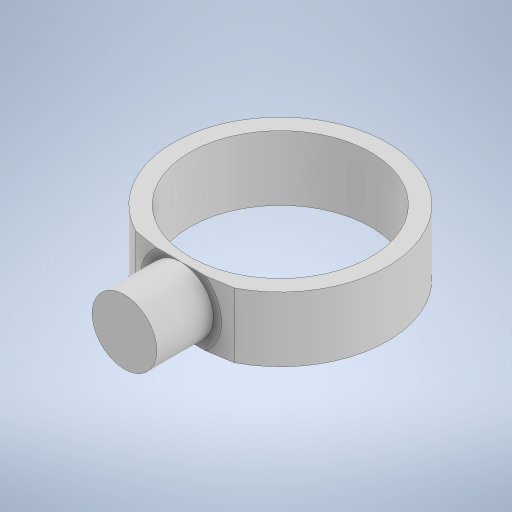
# Autodesk Inventor part: borde libre
Saved by Autodesk Inventor 2024 (Build 280153000, 153)
## iProperties
Created: 2024-04-03
Part Number: borde libre
Material: Generic
Document SubType Name: Modeling
Designer: compu
Density: 1 g/cm^3
Appearance: Default
Author: compu
Autodesk Inventor part; units mm, degrees
ref_plane "YZ Plane" through (0, 0, 0) normal (1, 0, 0) x (0, 1, 0)
ref_plane "XZ Plane" through (0, 0, 0) normal (0, 1, 0) x (-1, 0, 0)
ref_plane "XY Plane" through (0, 0, 0) normal (0, 0, 1) x (1, 0, 0)
sketch "Sketch1" plane through (0, 0, 0) normal (0, 1, 0) x (-1, 0, 0)
  line L0 (0, -18.55) -> (0, 18.55) projected
  line L1 (18.55, 0) -> (-18.55, 0) projected
  circle A0 centre (0, 0) radius 4
  circle A1 centre (0, 0) radius 11.2
  circle A2 centre (0, 0) radius 13.25
  line L2 (5, 12.2704) -> (-5, 12.2704)
  line L3 (6.0844, 11.7704) -> (-6.0844, 11.7704)
  dimension "d0" = 8
  dimension "d1" = 22.4
  dimension "d2" = 26.5
  dimension "d3" = 10
  dimension "d4" = 2.05
  dimension "d5" = 0.5
  constraints: 4 end point, 4 point on circle, 3 centre point, 3 coincident, 1 horizontal, 1 parallel
  measures "d0" diameter of A0
  measures "d1" diameter of A1
  measures "d2" diameter of A2
  measures "d3" distance of L2.start L2.end
  measures "d4" radial gap between concentric circles of A2 A1
  measures "d5" distance between parallel lines of L3 L2
extrude "Extrusion1" add sketch "Sketch1" along normal blind 8 contours A2 L1 A1 L0 | L0 A1 L1 A2 | A2 L3 L0 A1 L1 | L1 A1 L0 L3 A2
ref_plane "Work Plane1" through (6.0844, 0, 11.7704) normal (0, 0, 1) x (1, 0, 0)
sketch "Sketch2" plane through (6.0844, 0, 11.7704) normal (0, 0, 1) x (1, 0, 0)
  line L0 (-12.1689, 0) -> (0, 0) projected
  line L1 (0, 0) -> (0, 8) projected
  line L2 (-12.1689, 8) -> (0, 8) projected
  line L3 (-12.1689, 0) -> (-12.1689, 8) projected
  line L4 (-6.0844, -4.4) -> (-6.0844, 12.4) projected
  circle A0 centre (-6.0844, 4) radius 5
  point P0 (-6.0844, 0)
  point P1 (-9.0844, 8)
  point P2 (-9.0844, 0)
  point P3 (-3.0844, 0)
  point P4 (-3.0844, 8)
  dimension "d8" = 10
  dimension "d9" = 4
  constraints: 1 centre point, 1 midpoint
  measures "d8" diameter of A0
  measures "d9" distance from line of L0 A0.centre
extrude "Extrusion2" add sketch "Sketch2" along normal blind 0.5 contours A0 L2 L4 L0 | L4 L2 A0 L0
sketch "Sketch3" plane through (6.0844, 0, 12.2704) normal (0, 0, 1) x (1, 0, 0)
  line L0 (-9.0844, 0) -> (-3.0844, 0) projected
  arc A0 (-3.0844, 0) -> (-3.0844, 8) centre (-6.0844, 4) ccw projected
  line L1 (-3.0844, 8) -> (-9.0844, 8) projected
  arc A1 (-9.0844, 8) -> (-9.0844, 0) centre (-6.0844, 4) ccw projected
  circle A2 centre (-6.0844, 4) radius 4
  point P0 (-6.0844, 0)
  point P1 (-6.0844, 8)
  point P2 (-9.7017, 7)
  point P3 (-6.0844, 0)
  point P4 (-5.8287, 0)
  dimension "d12" = 8
  constraints: 1 centre point, 1 coincident
  measures "d12" diameter of A2
extrude "Extrusion3" add sketch "Sketch3" along normal blind 7 contours A2
loft "Loft1" add section 1 edges at (-4, 4, 12.2704) (-1.5, 8, 12.2704) (-5, 4, 12.2704) (-1.5, 0, 12.2704) section 2 edges at (-5, 4, 11.7704) (-4.5422, 8, 11.7704) (-6.0844, 4, 11.7704) (-4.5422, 0, 11.7704)
loft "Loft2" add section 1 edges at (2.8284, 6.8284, 12.2704) (2.8284, 1.1716, 12.2704) (1.5, 0, 12.2704) (5, 4, 12.2704) (1.5, 8, 12.2704) section 2 edges at (5, 4, 11.7704) (4.5422, 0, 11.7704) (6.0844, 4, 11.7704) (4.5422, 8, 11.7704)
body "Solid1"
